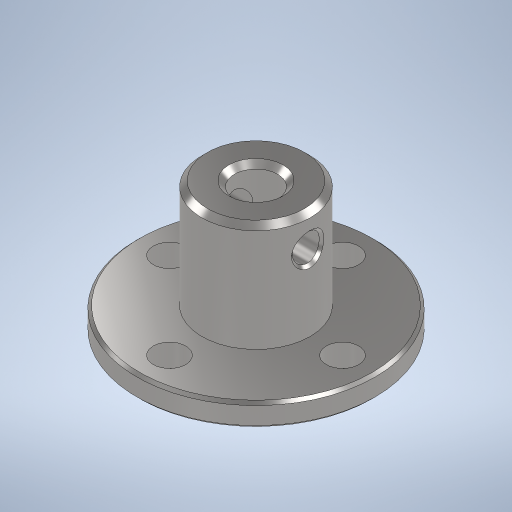
# Autodesk Inventor part: Hubs - 4mm
Saved by Autodesk Inventor 2023.4 (Build 274418000, 418)
## iProperties
Created: 2024-05-11
Part Number: Hubs - 4mm
Material: Stainless Steel
Document SubType Name: Modeling
Designer: Nathan Cai
Density: 8 g/cm^3
Appearance: Semi-Polished
Author: Nathan Cai
Autodesk Inventor part; units mm, degrees
ref_plane "YZ Plane" through (0, 0, 0) normal (1, 0, 0) x (0, 1, 0)
ref_plane "XZ Plane" through (0, 0, 0) normal (0, 1, 0) x (-1, 0, 0)
ref_plane "XY Plane" through (0, 0, 0) normal (0, 0, 1) x (1, 0, 0)
sketch "Sketch1" plane through (0, 0, 0) normal (0, 0, 1) x (1, 0, 0)
  line L0 (0, 0) -> (11, 0)
  line L1 (11, 0) -> (11, 2.1)
  line L2 (11, 2.1) -> (0, 2.1)
  line L3 (0, 2.1) -> (0, 0)
  line L4 (0, 0) -> (5, 0)
  line L5 (5, 0) -> (5, 12.1)
  line L6 (5, 12.1) -> (0, 12.1)
  line L7 (0, 12.1) -> (0, 0)
  line L8 (0, 12.1) -> (2, 12.1)
  line L9 (2, 12.1) -> (2, 0)
  line L10 (2, 0) -> (0, 0)
  line L11 (0, 0) -> (0, 12.1)
  point P0 (2, 0)
  point P1 (5, 2.1)
  dimension "d0" = 11
  dimension "d1" = 2.1
  dimension "d2" = 5
  dimension "d3" = 12.1
  dimension "d4" = 2
  constraints: 24 end point, 6 parallel, 3 horizontal, 3 perpendicular, 1 point on line
  measures "d0" distance of L2.end L1.end
  measures "d1" distance of L1.end L0.end
  measures "d2" distance of L6.end L5.end
  measures "d3" distance of L5.end L4.end
  measures "d4" distance of L9.end L10.end
revolve "Revolution1" add sketch "Sketch1" angle 360 about axis through (0, 12.1, 0) along (0, -1, 0) contours L9 L2 L5 L0 | L5 L2 L1 L0 | L9 L6 L5 L2
sketch "Sketch2" plane through (0, 0, 0) normal (0, -1, 0) x (1, 0, 0)
  circle A0 centre (0, 0) radius 8 construction
  line L0 (0, 0) -> (8, 0) construction
  circle A1 centre (8, 0) radius 1.5
  circle A2 centre (0, 8) radius 1.5
  circle A3 centre (-8, 0) radius 1.5
  circle A4 centre (0, -8) radius 1.5
  dimension "d6" = 16
  dimension "d7" = 3
  dimension "d10" = 360
  constraints: 4 centre point, 2 coincident, 2 end point, 1 horizontal, 1 horizontal alignment, 11 other
  measures "d7" diameter of A1
extrude "Extrusion1" cut sketch "Sketch2" against normal through all
sketch "Sketch3" plane through (0, 0, 0) normal (1, 0, 0) x (0, 1, 0)
  line L0 (12.1, 5) -> (12.1, -5) projected
  line L1 (12.1, 0) -> (0, 0) construction
  circle A0 centre (9.1, 0) radius 1.25
  dimension "d14" = 2.5
  dimension "d15" = 3
  constraints: 2 end point, 1 centre point, 1 horizontal, 1 midpoint, 1 point on line
  measures "d14" diameter of A0
  measures "d15" distance from line of L0 A0.centre
extrude "Extrusion2" cut sketch "Sketch3" along normal through all both and the other way through all
chamfer "Chamfer1" distance 0.5 angle 45 2 edges at (-5, 12.1, 0) (-2, 12.1, 0)
chamfer "Chamfer2" distance 0.25 angle 45 5 edges at (-11, 0, 0) (-11, 2.1, 0) (4.8412, 9.0999, -1.25) (4.8412, 9.1, 1.25) (-5, 7.85, -0.0003)
body "Solid1"
